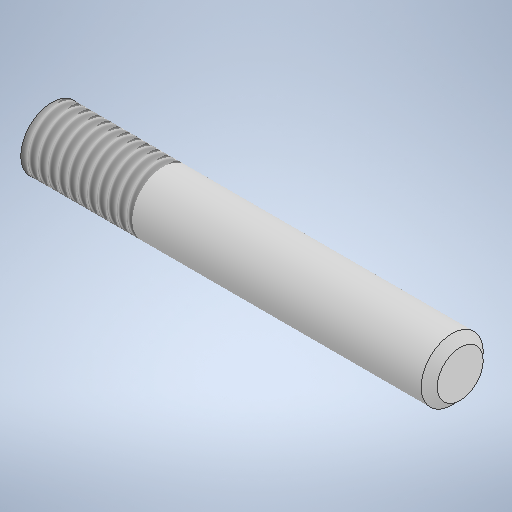
# Autodesk Inventor part: 207 part 1
Saved by Autodesk Inventor 2025.1 (Build 291241000, 241)
## iProperties
Created: 2024-08-23
Part Number: 207 part 1
Material: Generisch
Document SubType Name: Modeling
Designer: ffogue
Density: 1 g/cm^3
Appearance: Vorgabe
Author: ffogue
Autodesk Inventor part; units mm, degrees
ref_plane "YZ Plane" through (0, 0, 0) normal (1, 0, 0) x (0, 1, 0)
ref_plane "XZ Plane" through (0, 0, 0) normal (0, 1, 0) x (-1, 0, 0)
ref_plane "XY Plane" through (0, 0, 0) normal (0, 0, 1) x (1, 0, 0)
sketch "Sketch1" plane through (0, 0, 0) normal (0, 0, 1) x (1, 0, 0)
  line L0 (0, 0) -> (0, 2.5)
  line L1 (0, 2.5) -> (33, 2.5)
  line L2 (33, 2.5) -> (33, 0)
  line L3 (33, 0) -> (0, 0)
  dimension "d0" = 33
  dimension "d1" = 5
  constraints: 8 end point, 3 perpendicular, 1 vertical
  measures "d0" distance of L2.end L0.start
  measures "d1" diameter of L1 L3
revolve "Revolution1" add sketch "Sketch1" angle 360 about axis through (33, 0, 0) along (-1, 0, 0)
thread "Thread1" size "M5x0.8" class "6g" standard "ISO Metric profile" length 9
chamfer "Chamfer1" distance 0.65 angle 45 1 edges at (33, -2.5, 0)
body "Solid1"
